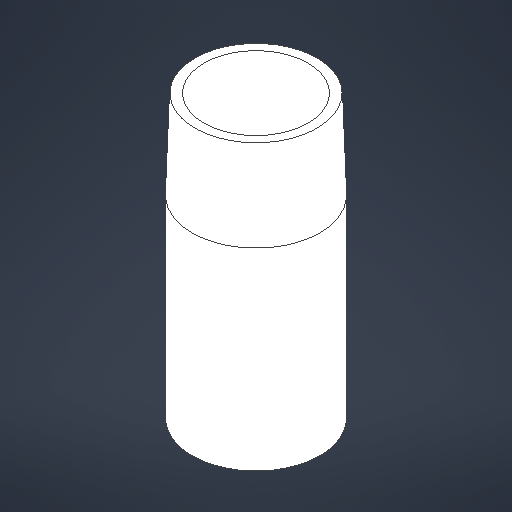
# Autodesk Inventor part: Pieza42
Saved by Autodesk Inventor 2026.2 (Build 302298000, 298)
## iProperties
Created: 2026-01-02
Part Number: Pieza42
Material: Genérico
Document SubType Name: Modeling
Designer: vicho
Density: 1 g/cm^3
Appearance: Valor por defecto
Author: vicho
Autodesk Inventor part; units mm, degrees
ref_plane "YZ Plane" through (0, 0, 0) normal (1, 0, 0) x (0, 1, 0)
ref_plane "XZ Plane" through (0, 0, 0) normal (0, 1, 0) x (-1, 0, 0)
ref_plane "XY Plane" through (0, 0, 0) normal (0, 0, 1) x (1, 0, 0)
sketch "Boceto1" plane through (0, 0, 0) normal (0, 0, 1) x (1, 0, 0)
  line L0 (0, 132.9544) -> (0, -187.2356) construction
  line L1 (-210.4029, 0) -> (220.8608, 0) construction
  line L2 (0, 47.5) -> (-20.5, 47.5)
  line L3 (0, -47.5) -> (-21.5, -47.5)
  line L4 (-21.5, -47.5) -> (-21.5, 65.7423) construction
  line L5 (-20.5, 47.5) -> (-21.5, 17.5)
  line L6 (-21.5, -47.5) -> (-21.5, 17.5)
  line L7 (0, 47.5) -> (0, -47.5)
  point P0 (0, 0)
  point P1 (-10.75, -47.5)
  point P2 (-10.25, 47.5)
  dimension "d0" = 20.5
  dimension "d1" = 21.5
  dimension "d2" = 95
  dimension "d3" = 30
  constraints: 16 end point, 5 point on line, 3 horizontal, 3 vertical, 2 midpoint, 1 collinear, 1 other
  measures "d0" distance of L2.end L2.start
  measures "d1" distance of L3.end L3.start
  measures "d2" vertical distance of point (-10.75, -47.5) point (-10.25, 47.5)
  measures "d3" distance from line of L5.end L2
revolve "Revolución1" add sketch "Boceto1" angle 360 about axis through (0, 132.9544, 0) along (0, -1, 0)
sketch "Boceto2" plane through (0, 47.5, 0) normal (0, 1, 0) x (1, 0, 0)
  circle A0 centre (0, 0) radius 17.5
  dimension "d5" = 35
  constraints: 1 centre point, 1 coincident
  measures "d5" diameter of A0
extrude "Extrusión1" cut sketch "Boceto2" against normal blind 150
